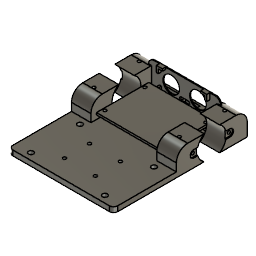
Master (Autodesk Fusion 360 design; units mm, degrees)
Autodesk Fusion 360 part; units mm, degrees
note: some values were not read from the file. Set by a fixed rule: which face or edge a step refers to.
sketch "Foundation" plane through (0, 0, 0) normal (0, 0, 1) x (1, 0, 0) in component "Plate"
  line L0 (0, 0) -> (102, 0)
  line L1 (102, 0) -> (102, 130)
  line L2 (102, 130) -> (0, 130)
  line L3 (0, 130) -> (0, 0)
  line L4 (24, 122) -> (38, 122)
  line L5 (38, 122) -> (38, 97)
  line L6 (38, 97) -> (24, 97)
  line L7 (24, 97) -> (24, 122)
  circle A0 centre (31, 104) radius 1.5
  line L8 (24, 104) -> (31, 104) construction
  line L9 (31, 104) -> (38, 104) construction
  line L10 (44, 97) -> (44, 122)
  line L11 (58, 122) -> (58, 97)
  line L12 (44, 104) -> (51, 104) construction
  line L13 (58, 97) -> (44, 97)
  line L14 (44, 122) -> (58, 122)
  circle A1 centre (51, 104) radius 1.5
  line L15 (51, 104) -> (58, 104) construction
  line L16 (64, 97) -> (64, 122)
  line L17 (78, 122) -> (78, 97)
  line L18 (64, 104) -> (71, 104) construction
  line L19 (78, 97) -> (64, 97)
  line L20 (64, 122) -> (78, 122)
  circle A2 centre (71, 104) radius 1.5
  line L21 (71, 104) -> (78, 104) construction
  line L22 (51, 104) -> (51, 130) construction
  circle A3 centre (15.075, 54.325) radius 3
  circle A4 centre (86.925, 54.325) radius 3
  circle A5 centre (15.075, 6.575) radius 3
  circle A6 centre (86.925, 6.575) radius 3
  line L23 (51, 6.575) -> (51, 0) construction
  circle A7 centre (15.075, 54.325) radius 2.45
  circle A8 centre (86.925, 54.325) radius 2.45
  circle A9 centre (15.075, 6.575) radius 2.45
  circle A10 centre (86.925, 6.575) radius 2.45
  circle A11 centre (36, 42.65) radius 1.55
  line L24 (86.925, 54.325) -> (86.925, 6.575) construction
  line L25 (38, 122) -> (24, 122)
  line L26 (24, 122) -> (24, 128)
  line L27 (24, 128) -> (38, 128)
  line L28 (38, 128) -> (38, 122)
  line L29 (44, 122) -> (44, 128)
  line L30 (58, 128) -> (58, 122)
  line L31 (44, 128) -> (58, 128)
  line L32 (64, 122) -> (64, 128)
  line L33 (78, 128) -> (78, 122)
  line L34 (64, 128) -> (78, 128)
  line L35 (15.075, 54.325) -> (86.925, 54.325) construction
  line L36 (15.075, 6.575) -> (86.925, 6.575) construction
  circle A12 centre (66, 42.65) radius 1.55
  circle A13 centre (36, 18.25) radius 1.55
  circle A14 centre (66, 18.25) radius 1.55
  line L37 (36, 18.25) -> (66, 18.25) construction
  line L38 (51, 18.25) -> (51, 6.575) construction
  line L39 (66, 42.65) -> (66, 18.25) construction
  line L40 (66, 30.45) -> (86.925, 30.45) construction
  line L41 (24, 97) -> (38, 97)
  line L42 (38, 97) -> (38, 87)
  line L43 (38, 87) -> (24, 87)
  line L44 (24, 87) -> (24, 97)
  line L45 (58, 97) -> (58, 87)
  line L46 (58, 87) -> (44, 87)
  line L47 (44, 87) -> (44, 97)
  line L48 (78, 97) -> (78, 87)
  line L49 (78, 87) -> (64, 87)
  line L50 (64, 87) -> (64, 97)
  point P0 (51, 6.575)
  dimension "d30" = 3
  dimension "d31" = 7
  dimension "d32" = 25
  dimension "d33" = 14
  dimension "d36" = 20
  dimension "d37" = 0
  dimension "d38" = 102
  dimension "d39" = 130
  dimension "d51" = 6
  dimension "d54" = 71.85
  dimension "d55" = -47.75
  dimension "d56" = 4.9
  dimension "d61" = 3.1
  dimension "d109" = 6
  dimension "d110" = 2
  dimension "d124" = 30
  dimension "d125" = -24.4
  dimension "d130" = 6.575
  dimension "d151" = 10
  constraint horizontal L0
  constraint vertical L1
  constraint horizontal L2
  constraint vertical L3
  constraint coincident L0.start L3.end
  constraint horizontal L4
  constraint vertical L5
  constraint horizontal L6
  constraint vertical L7
  constraint coincident L7 L8.start
  constraint coincident A0.centre L8.end
  constraint coincident L5 L9.end
  constraint equal L8 L9
  constraint perpendicular L7 L8
  constraint perpendicular L5 L9
  constraint coincident L12.end A1.centre
  constraint midpoint L2 L22.end
  constraint perpendicular L2 L22
  constraint midpoint L0 L23.end
  constraint concentric A3 A7
  constraint coincident A4.centre A8.centre
  constraint coincident A6.centre A10.centre
  constraint coincident P0 L23.start
  constraint horizontal L25
  constraint vertical L26
  constraint horizontal L27
  constraint vertical L28
  constraint collinear L7 L26
  constraint coincident A3.centre A7.centre
  constraint coincident A5.centre A9.centre
  constraint midpoint P0 L36
  constraint perpendicular L23 L36
  constraint coincident A13.centre L37.start
  constraint coincident A14.centre L37.end
  constraint midpoint L37 L38.start
  constraint perpendicular L37 L38
  constraint coincident A12.centre L39.start
  constraint midpoint L39 L40.start
  constraint midpoint L24 L40.end
  constraint perpendicular L39 L40
  constraint horizontal L41
  constraint vertical L42
  constraint horizontal L43
  constraint vertical L44
  constraint collinear L5 L42
  measures "d30" diameter of A0
  measures "d31" distance of L6 A0.centre
  measures "d32" distance of L4.start L6.end
  measures "d33" distance of L5.end L6.end
  measures "d38" distance of L1.end L2.end
  measures "d39" distance of L0.start L2.end
  measures "d51" diameter of A3
  measures "d56" diameter of A7
  measures "d61" diameter of A11
  measures "d109" distance of L4.start L26.end
  measures "d110" distance of L2 L27
  measures "d130" distance of P0 L23.end
  measures "d151" distance of L6.end L43.end
extrude "Extrude1" add sketch "Foundation" along normal blind 5 contours L0 L1 L2 L3 | A3 | A4 | A5 | A6 makes body 1 in component "Plate"
extrude "Extrude2" add sketch "Foundation" along normal blind 1 contours L4 L5 L6 L7 L25 L41 | L10 L11 L13 L14 | L16 L17 L19 L20 bodies 1 in component "Plate"
extrude "Extrude13" add sketch "Foundation" along normal blind 3 contours L6 L41 L42 L43 L44 | L13 L45 L46 L47 | L19 L48 L49 L50 bodies 1 in component "Plate"
chamfer "Chamfer1" distance 2 angle 45 3 edges at (71, 87, 5) (51, 87, 5) (31, 87, 5) measured on face at (48.6667, 58.3282, 5) measured on face at (48.6667, 58.3282, 5) measured on face at (48.6667, 58.3282, 5) on bodies 1 in component "Plate"
extrude "Extrude4" cut sketch "Foundation" along normal blind 1.8 contours A3 | A4 | A5 | A6 bodies 1 in component "Plate"
sketch "MotorHolder" plane through (0, 0, 0) normal (-1, 0, 0) x (0, -1, 0) in component "Plate"
  line L0 (-130, 0) -> (0, 0)
  line L1 (0, 0) -> (0, 5)
  line L2 (0, 5) -> (-130, 5)
  line L3 (-130, 5) -> (-130, 0)
  circle A0 centre (-95.5, 11.8216) radius 14
  line L4 (-119, 23.6432) -> (-72, 23.6432)
  line L5 (-72, 23.6432) -> (-72, 0)
  line L6 (-72, 0) -> (-119, 0)
  line L7 (-119, 0) -> (-119, 23.6432)
  line L8 (-95.5, 11.8216) -> (-95.5, 23.6432) construction
  circle A1 centre (-113, 11.8216) radius 1.5
  line L9 (-113, 11.8216) -> (-119, 11.8216) construction
  line L10 (-109.0554, 15.3216) -> (-113, 15.3216)
  arc A2 (-113, 15.3216) -> (-113, 8.3216) centre (-113, 11.8216) ccw
  line L11 (-113, 8.3216) -> (-109.0554, 8.3216)
  line L12 (-81.9446, 15.3216) -> (-78, 15.3216)
  arc A3 (-78, 8.3216) -> (-78, 15.3216) centre (-78, 11.8216) ccw
  circle A4 centre (-78, 11.8216) radius 1.5
  line L13 (-78, 8.3216) -> (-81.9446, 8.3216)
  line L14 (-130, 5) -> (-130, 12.6432)
  arc A5 (-119, 23.6432) -> (-130, 12.6432) centre (-119, 12.6432) ccw
  arc A6 (-61, 12.6432) -> (-72, 23.6432) centre (-72, 12.6432) ccw
  line L15 (-61, 5) -> (-61, 12.6432)
  point P0 (-103, 23.6432)
  point P1 (-88, 23.6432)
  point P2 (-103, 0)
  point P3 (-88, 0)
  dimension "d72" = 28
  dimension "d73" = 3
  dimension "d74" = 17.5
  dimension "d75" = 15
  dimension "d76" = 6
  dimension "d77" = 15
  dimension "d78" = 3.5
  dimension "d80" = 11
  constraint horizontal L4
  constraint vertical L5
  constraint horizontal L6
  constraint vertical L7
  constraint coincident A0.centre L8.start
  constraint midpoint L4 L8.end
  constraint perpendicular L4 L8
  constraint coincident A1.centre L9.start
  constraint midpoint L7 L9.end
  constraint perpendicular L7 L9
  constraint coincident A0 P0
  constraint coincident L4 P0
  constraint coincident L4 P1
  constraint coincident A0 P1
  constraint coincident A0 P2
  constraint coincident L6 P2
  constraint coincident A0 P3
  constraint coincident L6 P3
  constraint coincident A0 L10.start
  constraint perpendicular L7 L10
  constraint tangent L10 A2
  constraint coincident A0 L11.end
  constraint tangent A2 L11
  constraint parallel L9 L11
  constraint symmetric L8 A1 A4
  constraint symmetric L8 L10.start L12.start
  constraint symmetric L8 L10.end L12.end
  constraint symmetric L8 A2.end A3.start
  constraint symmetric L8 A2 A3
  constraint symmetric L8 L11.end L13.end
  constraint collinear L0 L6
  constraint coincident L2.end L3.start
  constraint perpendicular L2 L14
  constraint tangent L14 A5
  constraint coincident L7 A5.centre
  constraint symmetric L4.start L8 L4.end
  constraint symmetric L8 L2.end L15.start
  constraint symmetric L8 L14.end A6.start
  constraint symmetric L8 A5 A6
  measures "d72" diameter of A0
  measures "d73" diameter of A1
  measures "d74" horizontal distance of A0.centre A1.centre
  measures "d75" distance of P0 P1
  measures "d76" distance of L7 A1.centre
  measures "d77" distance of P2 P3
  measures "d78" radius of A2
  measures "d80" distance of L3 L7
extrude "Extrude7" add sketch "MotorHolder" against normal blind 19 contours L2 L7 L14 A5 | L2 A0 L4 L7 L10 A2 L11 | L2 A0 L4 L5 L12 A3 L13 | A0 L10 A2 L11 | L2 L5 A6 L15 | A0 L12 A3 L13 | A1 | A4 bodies 1 in component "Plate"
extrude "Extrude8" cut sketch "MotorHolder" against normal up to surface (19 mm away) contours L0 L2 A0 L6 bodies 1 in component "Plate"
extrude "Extrude9" cut sketch "MotorHolder" against normal blind 1 contours A0 L10 A2 L11 | A0 L12 A3 L13 | A1 | A4 bodies 1 in component "Plate"
extrude "Extrude12" cut sketch "MotorHolder" against normal blind 5 contours A1 | A4 bodies 1 in component "Plate"
ref_plane "WorkPlane1" through (51, 65, 11.8216) normal (-1, 0, 0) x (0, -1, 0) in component "Plate"
mirror "Mirror1" about plane through (51, 65, 11.8216) normal (-1, 0, 0) of "Extrude7", "Extrude8", "Extrude9", "Extrude12" in component "Plate"
ref_plane "WorkPlane1" through (51, 121, 6.3216) normal (0, 1, 0) x (-1, 0, 0) in component "UltrasonicHolder"
sketch "Sketch1" plane through (0, 121, 0) normal (0, 1, 0) x (1, 0, 0) in component "UltrasonicHolder"
  circle A0 centre (64, -17) radius 8
  circle A1 centre (38, -17) radius 8
  line L0 (80.6432, -29) -> (21.3568, -29)
  line L1 (16, -23.6432) -> (16, -5)
  line L2 (16, -5) -> (86, -5)
  line L3 (86, -5) -> (86, -23.6432)
  line L4 (64, -17) -> (38, -17) construction
  line L5 (51, -17) -> (51, -5) construction
  line L6 (54.25, -11.5) -> (47.75, -11.5)
  arc A2 (47.75, -8) -> (47.75, -11.5) centre (47.75, -9.75) ccw
  line L7 (47.75, -8) -> (54.25, -8)
  arc A3 (54.25, -11.5) -> (54.25, -8) centre (54.25, -9.75) ccw
  line L8 (64, -9) -> (38, -9) construction
  line L9 (102, 0) -> (0, 0)
  line L10 (0, 0) -> (0, -12.6432)
  line L11 (0, -12.6432) -> (19, -12.6432)
  line L12 (19, -12.6432) -> (19, -5)
  line L13 (19, -5) -> (83, -5)
  line L14 (83, -5) -> (83, -12.6432)
  line L15 (83, -12.6432) -> (102, -12.6432)
  line L16 (102, -12.6432) -> (102, 0)
  line L17 (102, -12.6432) -> (102, -23.6432)
  line L18 (102, -12.6432) -> (83, -12.6432)
  line L19 (83, -23.6432) -> (83, -12.6432)
  line L20 (83, -23.6432) -> (102, -23.6432)
  line L21 (0, -12.6432) -> (0, -23.6432)
  line L22 (0, -23.6432) -> (19, -23.6432)
  line L23 (19, -23.6432) -> (19, -12.6432)
  line L24 (19, -12.6432) -> (0, -12.6432)
  line L25 (75.5, -29) -> (69.5, -29)
  line L26 (69.5, -29) -> (69.5, -27)
  line L27 (69.5, -27) -> (73.5, -27)
  line L28 (73.5, -27) -> (73.5, -23)
  line L29 (73.5, -23) -> (75.5, -23)
  line L30 (75.5, -23) -> (75.5, -29)
  line L31 (26.5, -23) -> (26.5, -29)
  line L32 (26.5, -29) -> (32.5, -29)
  line L33 (32.5, -29) -> (32.5, -27)
  line L34 (32.5, -27) -> (28.5, -27)
  line L35 (28.5, -27) -> (28.5, -23)
  line L36 (28.5, -23) -> (26.5, -23)
  line L37 (69.5, -7) -> (73.5, -7)
  line L38 (75.5, -5) -> (69.5, -5)
  line L39 (75.5, -11) -> (75.5, -5)
  line L40 (69.5, -5) -> (69.5, -7)
  line L41 (73.5, -7) -> (73.5, -11)
  line L42 (73.5, -11) -> (75.5, -11)
  line L43 (32.5, -7) -> (28.5, -7)
  line L44 (28.5, -7) -> (28.5, -11)
  line L45 (32.5, -5) -> (32.5, -7)
  line L46 (28.5, -11) -> (26.5, -11)
  line L47 (26.5, -5) -> (32.5, -5)
  line L48 (26.5, -11) -> (26.5, -5)
  arc A4 (80.6432, -29) -> (86, -23.6432) centre (80.6432, -23.6432) ccw
  arc A5 (16, -23.6432) -> (21.3568, -29) centre (21.3568, -23.6432) ccw
  point P0 (56, -9.75)
  point P1 (46, -9.75)
  point P2 (51, -11.5)
  point P3 (86, -23.6432)
  dimension "d94" = 16
  dimension "d98" = -26
  dimension "d99" = 0
  dimension "d100" = 10
  dimension "d101" = 3.5
  dimension "d103" = 1
  dimension "d106" = 3
  dimension "d111" = 2
  dimension "d113" = 4
  dimension "d114" = 22.5
  dimension "d117" = 24
  constraint horizontal L0
  constraint vertical L1
  constraint horizontal L2
  constraint vertical L3
  constraint coincident A0.centre L4.start
  constraint coincident A1.centre L4.end
  constraint midpoint L4 L5.start
  constraint midpoint L2 L5.end
  constraint perpendicular L2 L5
  constraint horizontal L6
  constraint tangent L6 A2
  constraint tangent A2 L7
  constraint perpendicular L5 L7
  constraint tangent L7 A3
  constraint tangent L6 A3
  constraint midpoint A3 P0
  constraint midpoint A2 P1
  constraint midpoint L6 P2
  constraint coincident L5 P2
  constraint coincident A0 L8.start
  constraint coincident A1 L8.end
  constraint tangent A1 L8
  constraint tangent A0 L8
  constraint symmetric L5 L19 L23
  constraint collinear L2 L13
  constraint horizontal L25
  constraint perpendicular L25 L26
  constraint perpendicular L26 L27
  constraint perpendicular L27 L28
  constraint perpendicular L28 L29
  constraint perpendicular L25 L30
  constraint equal L26 L29
  constraint equal L25 L30
  constraint collinear L0 L25
  constraint symmetric L5 L25.start L31.end
  constraint symmetric L5 L25.end L32.end
  constraint symmetric L5 L26.end L33.end
  constraint symmetric L5 L27.end L34.end
  constraint symmetric L5 L28.end L35.end
  constraint symmetric L5 L29.end L31.start
  constraint symmetric L4 L25.start L38.start
  constraint symmetric L4 L25.end L38.end
  constraint symmetric L4 L26.end L37.start
  constraint symmetric L4 L27.end L37.end
  constraint symmetric L4 L28.end L41.end
  constraint symmetric L4 L29.end L39.start
  constraint symmetric L4 L31.start L46.end
  constraint symmetric L4 L31.end L47.start
  constraint symmetric L4 L32.end L45.start
  constraint symmetric L4 L33.end L43.start
  constraint symmetric L4 L34.end L43.end
  constraint symmetric L4 L35.end L44.end
  constraint coincident L3 P3
  constraint coincident L20 P3
  constraint coincident L3.end A4.end
  constraint tangent L3 A4
  constraint tangent L0 A4
  constraint coincident L1.start L22
  constraint tangent L0 A5
  constraint tangent L1 A5
  measures "d94" diameter of A0
  measures "d100" distance of P0 P1
  measures "d101" distance of L6 L7
  measures "d103" distance of L7 L8
  measures "d106" distance of L3 L19
  measures "d111" distance of L28.end L29.end
  measures "d113" distance of L27.end L28.end
  measures "d114" distance of L5 L28
  measures "d117" distance of L0 L2
extrude "Extrude1'" add sketch "Sketch1" against normal blind 1 separate body contours L0 L2 L12 L13 L14 L19 L20 L22 L23 L26 L27 L28 L29 L30 L31 L33 L34 L35 L36 L37 L39 L40 L41 L42 L43 L44 L45 L46 L48 A4 A5 | L0 L25 L26 L27 L28 L29 L30 | L3 L15 L18 L19 L20 | L2 L3 L14 L15 L18 | L0 L31 L32 L33 L34 L35 L36 | L2 L13 L37 L38 L39 L40 L41 L42 | L1 L11 L22 L23 L24 | L1 L2 L11 L12 L24 | L2 L13 L43 L44 L45 L46 L47 L48 makes body 2 in component "UltrasonicHolder"
extrude "Extrude2'" add sketch "Sketch1" against normal blind 4 contours L0 L25 L26 L27 L28 L29 L30 | L0 L31 L32 L33 L34 L35 L36 | L2 L13 L37 L38 L39 L40 L41 L42 | L2 L13 L43 L44 L45 L46 L47 L48 bodies 2 in component "UltrasonicHolder"
combine "Combine1" operation cut target body 1 tool bodies 2 keep tools in component "Plate"
fillet "Fillet1" radius 4 2 edges at (0, 0, 2.5) (102, 0, 2.5) on bodies 1 in component "Plate"
sketch "SupportHoles" plane through (0, 0, 5) normal (0, 0, 1) x (-1, 0, 0) in component "Plate"
  arc A0 (-98, 0) -> (-102, -4) centre (-98, -4) ccw
  line L0 (-102, -4) -> (-102, -61)
  line L1 (-102, -61) -> (-83, -61)
  line L2 (-83, -61) -> (-83, -83.2744)
  line L3 (0, -61) -> (0, -4)
  arc A1 (0, -4) -> (-4, 0) centre (-4, -4) ccw
  line L4 (-4, 0) -> (-98, 0)
  circle A2 centre (-15.075, -6.575) radius 2.45
  circle A3 centre (-66, -42.65) radius 1.55
  circle A4 centre (-36, -18.25) radius 1.55
  circle A5 centre (-66, -18.25) radius 1.55
  circle A6 centre (-36, -42.65) radius 1.55
  circle A7 centre (-86.925, -6.575) radius 2.45
  line L5 (-26.75, -73.6372) -> (-28.25, -73.6372)
  line L6 (-28.25, -73.6372) -> (-28.25, -70.6372)
  line L7 (-28.25, -70.6372) -> (-26.75, -70.6372)
  line L8 (-26.75, -70.6372) -> (-26.75, -73.6372)
  line L9 (-83, -61) -> (-83, -83.2744)
  line L10 (-19, -83.2744) -> (-19, -61)
  line L11 (-19, -72.1372) -> (-83, -72.1372) construction
  line L12 (-27.5, -97) -> (-27.5, -73.6372) construction
  line L13 (-31, -97) -> (-31, -72.1372) construction
  line L14 (-35.25, -70.6372) -> (-35.25, -73.6372)
  line L15 (-35.25, -73.6372) -> (-33.75, -73.6372)
  line L16 (-33.75, -70.6372) -> (-35.25, -70.6372)
  line L17 (-33.75, -73.6372) -> (-33.75, -70.6372)
  line L18 (-46.75, -70.6372) -> (-46.75, -73.6372)
  line L19 (-46.75, -73.6372) -> (-48.25, -73.6372)
  line L20 (-48.25, -73.6372) -> (-48.25, -70.6372)
  line L21 (-48.25, -70.6372) -> (-46.75, -70.6372)
  line L22 (-53.75, -73.6372) -> (-53.75, -70.6372)
  line L23 (-55.25, -73.6372) -> (-53.75, -73.6372)
  line L24 (-55.25, -70.6372) -> (-55.25, -73.6372)
  line L25 (-53.75, -70.6372) -> (-55.25, -70.6372)
  line L26 (-66.75, -70.6372) -> (-66.75, -73.6372)
  line L27 (-66.75, -73.6372) -> (-68.25, -73.6372)
  line L28 (-68.25, -73.6372) -> (-68.25, -70.6372)
  line L29 (-68.25, -70.6372) -> (-66.75, -70.6372)
  line L30 (-73.75, -73.6372) -> (-73.75, -70.6372)
  line L31 (-75.25, -73.6372) -> (-73.75, -73.6372)
  line L32 (-75.25, -70.6372) -> (-75.25, -73.6372)
  line L33 (-73.75, -70.6372) -> (-75.25, -70.6372)
  circle A8 centre (-21.5, -72.1372) radius 1.5
  circle A9 centre (-21.5, -111) radius 1.5
  line L34 (-19, -111) -> (-24, -111) construction
  line L35 (-24, -85) -> (-24, -128)
  line L36 (-21.5, -111) -> (-21.5, -72.1372) construction
  line L37 (-51, -97) -> (-51, -72.1372) construction
  circle A10 centre (-80.5, -111) radius 1.5
  circle A11 centre (-80.5, -72.1372) radius 1.5
  circle A12 centre (-86.925, -54.325) radius 2.45
  circle A13 centre (-15.075, -54.325) radius 2.45
  line L38 (-19, -119) -> (-19, -103)
  line L39 (-19, -88) -> (-19, -72)
  line L40 (-58, -85) -> (-44, -85)
  line L41 (-78, -85) -> (-64, -85)
  line L42 (-38, -85) -> (-24, -85)
  line L43 (-38, -97) -> (-24, -97)
  line L44 (-58, -97) -> (-44, -97)
  line L45 (-31, -97) -> (-24, -97) construction
  point P0 (-26.75, -72.1372)
  point P1 (-31, -97)
  point P2 (-27.5, -97)
  point P3 (-34.5, -73.6372)
  point P4 (-35.25, -72.1372)
  dimension "d131" = 3
  dimension "d132" = 1.5
  dimension "d135" = -20
  dimension "d136" = 0
  dimension "d139" = 3
  dimension "d140" = 3
  constraint horizontal L5
  constraint vertical L6
  constraint horizontal L7
  constraint vertical L8
  constraint midpoint L10 L11.start
  constraint midpoint L9 L11.end
  constraint midpoint L8 P0
  constraint coincident L11 P0
  constraint midpoint L5 L12.end
  constraint perpendicular L5 L12
  constraint coincident P1 L13.start
  constraint coincident L11 L13.end
  constraint perpendicular L11 L13
  constraint symmetric L5.start L13 L14.end
  constraint symmetric L5.end L13 L15.end
  constraint symmetric L6.end L13 L16.start
  constraint symmetric L7.end L13 L14.start
  constraint symmetric P0 L13 P4
  constraint symmetric L12.end L13 P3
  constraint coincident L11 A8.centre
  constraint coincident L34.end L35
  constraint perpendicular L34 L35
  constraint midpoint A9.centre L34
  constraint coincident A9.centre L36.start
  constraint coincident A8.centre L36.end
  constraint perpendicular L11 L36
  constraint midpoint L11 L37.end
  constraint symmetric A8 L37 A11
  constraint symmetric A9 L37 A10
  constraint midpoint L34.start L38
  constraint vertical L37
  constraint midpoint L37.start L44
  constraint midpoint P1 L43
  constraint coincident L43.end L45.end
  constraint midpoint P2 L45
  constraint coincident P2 L12.start
  measures "d131" distance of L5.start L7.end
  measures "d132" distance of L6.end L7.end
  measures "d139" diameter of A8
  measures "d140" diameter of A9
extrude "Extrude10" cut sketch "SupportHoles" against normal up to surface (5 mm away) contours L5 L6 L7 L8 | L14 L15 L16 L17 | L18 L19 L20 L21 | L22 L23 L24 L25 | L26 L27 L28 L29 | L30 L31 L32 L33 | A8 | A9 | A10 | A11 bodies 1 in component "Plate"
ref_plane "WorkPlane1" through (51, 65, 9) normal (0, 0, 1) x (1, 0, 0) in component "SecondLayer"
sketch "Sketch1 (2)" plane through (0, 0, 9) normal (0, 0, 1) x (1, 0, 0) in component "SecondLayer"
  line L0 (64, 85) -> (64, 128)
  line L1 (64, 128) -> (78, 128)
  line L2 (78, 128) -> (78, 85)
  circle A0 centre (15.075, 54.325) radius 2.45
  circle A1 centre (66, 18.25) radius 1.55
  circle A2 centre (66, 42.65) radius 1.55
  circle A3 centre (86.925, 6.575) radius 2.45
  circle A4 centre (36, 18.25) radius 1.55
  circle A5 centre (36, 42.65) radius 1.55
  circle A6 centre (15.075, 6.575) radius 2.45
  circle A7 centre (86.925, 54.325) radius 2.45
  line L3 (38, 128) -> (38, 85)
  line L4 (24, 85) -> (24, 128)
  line L5 (24, 128) -> (38, 128)
  line L6 (58, 128) -> (58, 85)
  line L7 (44, 85) -> (44, 128)
  line L8 (44, 128) -> (58, 128)
  arc A8 (98, 0) -> (102, 4) centre (98, 4) ccw
  line L9 (102, 4) -> (102, 61)
  line L10 (102, 61) -> (83, 61)
  line L11 (83, 61) -> (83, 83.2744)
  line L12 (83, 83.2744) -> (83, 107.7256)
  line L13 (83, 107.7256) -> (83, 120)
  line L14 (83, 120) -> (86, 120)
  line L15 (86, 120) -> (86, 121)
  line L16 (86, 121) -> (83, 121)
  line L17 (83, 121) -> (83, 130)
  line L18 (83, 130) -> (19, 130)
  line L19 (19, 130) -> (19, 121)
  line L20 (19, 121) -> (16, 121)
  line L21 (16, 121) -> (16, 120)
  line L22 (16, 120) -> (19, 120)
  line L23 (19, 120) -> (19, 107.7256)
  line L24 (19, 107.7256) -> (19, 83.2744)
  line L25 (19, 83.2744) -> (19, 61)
  line L26 (19, 61) -> (0, 61)
  line L27 (0, 61) -> (0, 4)
  arc A9 (0, 4) -> (4, 0) centre (4, 4) ccw
  line L28 (4, 0) -> (98, 0)
  circle A10 centre (21.5, 72.1372) radius 1.5
  line L29 (73.75, 70.6372) -> (73.75, 73.6372)
  line L30 (73.75, 73.6372) -> (75.25, 73.6372)
  line L31 (75.25, 73.6372) -> (75.25, 70.6372)
  line L32 (75.25, 70.6372) -> (73.75, 70.6372)
  line L33 (33.75, 73.6372) -> (35.25, 73.6372)
  line L34 (35.25, 73.6372) -> (35.25, 70.6372)
  line L35 (35.25, 70.6372) -> (33.75, 70.6372)
  line L36 (33.75, 70.6372) -> (33.75, 73.6372)
  line L37 (48.25, 70.6372) -> (46.75, 70.6372)
  line L38 (46.75, 70.6372) -> (46.75, 73.6372)
  line L39 (46.75, 73.6372) -> (48.25, 73.6372)
  line L40 (48.25, 73.6372) -> (48.25, 70.6372)
  circle A11 centre (21.5, 111) radius 1.5
  circle A12 centre (80.5, 72.1372) radius 1.5
  line L41 (68.25, 70.6372) -> (66.75, 70.6372)
  line L42 (66.75, 70.6372) -> (66.75, 73.6372)
  line L43 (66.75, 73.6372) -> (68.25, 73.6372)
  line L44 (68.25, 73.6372) -> (68.25, 70.6372)
  line L45 (26.75, 70.6372) -> (26.75, 73.6372)
  line L46 (26.75, 73.6372) -> (28.25, 73.6372)
  line L47 (28.25, 73.6372) -> (28.25, 70.6372)
  line L48 (28.25, 70.6372) -> (26.75, 70.6372)
  line L49 (53.75, 70.6372) -> (53.75, 73.6372)
  line L50 (53.75, 73.6372) -> (55.25, 73.6372)
  line L51 (55.25, 73.6372) -> (55.25, 70.6372)
  line L52 (55.25, 70.6372) -> (53.75, 70.6372)
  circle A13 centre (80.5, 111) radius 1.5
  line L53 (75.5, 120) -> (80.6432, 120)
  line L54 (80.6432, 120) -> (80.6432, 121)
  line L55 (80.6432, 121) -> (21.3568, 121)
  line L56 (21.3568, 121) -> (21.3568, 120)
  line L57 (21.3568, 120) -> (26.5, 120)
  line L58 (26.5, 120) -> (26.5, 117)
  line L59 (26.5, 117) -> (32.5, 117)
  line L60 (32.5, 117) -> (32.5, 120)
  line L61 (32.5, 120) -> (69.5, 120)
  line L62 (69.5, 120) -> (69.5, 117)
  line L63 (69.5, 117) -> (75.5, 117)
  line L64 (75.5, 117) -> (75.5, 120)
  line L65 (19, 117) -> (83, 117)
  line L66 (83, 117) -> (83, 66.1372)
  line L67 (83, 66.1372) -> (19, 66.1372)
  line L68 (19, 66.1372) -> (19, 117)
  line L69 (21.5, 111) -> (21.5, 117) construction
  line L70 (21.5, 72.1372) -> (21.5, 66.1372) construction
  line L71 (38, 85) -> (24, 85)
  line L72 (78, 85) -> (64, 85)
  line L73 (58, 85) -> (44, 85)
  constraint coincident L13 L65.end
  constraint perpendicular L13 L65
  constraint coincident L11 L66.end
  constraint coincident L25 L67.end
  constraint perpendicular L25 L67
  constraint coincident L23 L65.start
  constraint collinear L59 L65
  constraint coincident A11.centre L69.start
  constraint coincident L65 L69.end
  constraint perpendicular L65 L69
  constraint coincident A10.centre L70.start
  constraint coincident L67 L70.end
  constraint perpendicular L67 L70
  constraint equal L69 L70
extrude "Extrude1''" add sketch "Sketch1 (2)" along normal blind 2 separate body contours L0 L2 L3 L4 L6 L7 L11 L12 L13 L23 L24 L25 L65 L66 L67 L68 L71 L72 L73 | L0 L2 L63 L65 L72 | L6 L7 L65 L73 | L3 L4 L59 L65 L71 | L29 L30 L31 L32 | L33 L34 L35 L36 | L37 L38 L39 L40 | L41 L42 L43 L44 | L45 L46 L47 L48 | L49 L50 L51 L52 makes body 3 in component "SecondLayer"
sketch "Sketch9" plane through (0, 0, 23.6432) normal (0, 0, 1) x (-1, 0, 0) in component "Plate"
  line L0 (0, -119) -> (0, -103)
  line L1 (0, -103) -> (-19, -103)
  line L2 (-19, -103) -> (-19, -119)
  line L3 (0, -88) -> (0, -72)
  line L4 (0, -72) -> (-19, -72)
  line L5 (-19, -72) -> (-19, -88)
  line L6 (-19, -88) -> (0, -88)
  line L7 (-102, -103) -> (-102, -119)
  line L8 (-102, -119) -> (-83, -119)
  line L9 (-83, -119) -> (-83, -103)
  line L10 (-83, -103) -> (-102, -103)
  line L11 (-102, -72) -> (-102, -88)
  line L12 (-102, -88) -> (-83, -88)
  line L13 (-83, -88) -> (-83, -72)
  line L14 (-83, -72) -> (-102, -72)
  circle A0 centre (-9.5, -117.5) radius 1.5
  line L15 (0, -119) -> (-19, -119) construction
  line L16 (-51, -96.7198) -> (-51, 23.7198)
  circle A1 centre (-92.5, -117.5) radius 1.5
  line L17 (0, -103) -> (0, -88) construction
  line L18 (-102, -103) -> (-102, -88) construction
  line L19 (0, -95.5) -> (-102, -95.5) construction
  circle A2 centre (-9.5, -73.5) radius 1.5
  circle A3 centre (-92.5, -73.5) radius 1.5
  point P0 (-9.5, -119)
  dimension "d146" = 3
  constraint coincident L0.start L15.start
  constraint coincident L2.end L15.end
  constraint midpoint L15 P0
  constraint coincident A0 P0
  constraint tangent A0 L15
  constraint symmetric A0 L16 A1
  constraint coincident L0.end L1.start
  constraint coincident L3.start L6.end
  constraint coincident L7.start L10.end
  constraint coincident L11.end L12.start
  constraint midpoint L17 L19.start
  constraint midpoint L18 L19.end
  constraint symmetric A0 L19 A2
  constraint symmetric A1 L19 A3
  measures "d146" diameter of A0
extrude "Extrude11" cut sketch "Sketch9" against normal blind 6 contours A2 | A1 | A3 | A0 bodies 1 in component "Plate"
move_face "OffsetFaces1" offset -0.1 4 faces at (85, 120, 11.1992) (85, 121, 11.1533) (18, 120, 11.1992) (17, 121, 17.3066) on bodies 1 in component "Plate"
move_face "OffsetFaces1'" offset -0.2 6 faces at (19, 113.9085, 9.6667) (19, 99.5752, 9.6667) (19, 77.562, 9.6667) (83, 71.8496, 9.6667) (83, 91.4248, 9.6667) (83, 110.8171, 10.3333) on bodies 3 in component "SecondLayer"
component "Plate" placed x (1, 0, 0) y (0, 1, 0) z (0, 0, 1) at (0, 0, 0)
component "UltrasonicHolder" placed x (1, 0, 0) y (0, 1, 0) z (0, 0, 1) at (0, 0, 0)
component "SecondLayer" placed x (1, 0, 0) y (0, 1, 0) z (0, 0, 1) at (0, 0, 0)
equation "Plate_Thickness = 8 mm"
equation "Pole_Height = 50 mm"
equation "Plate_Hole_Diameter = 6 mm"
equation "RPi_Hole_Diameter = 2.75 mm"
equation "d51 = Plate_Hole_Diameter"
equation "d77 = d75"
equation "d113 = 2 * d111"
equation "d114 = ( 45 / 2 ) * 1 mm"
